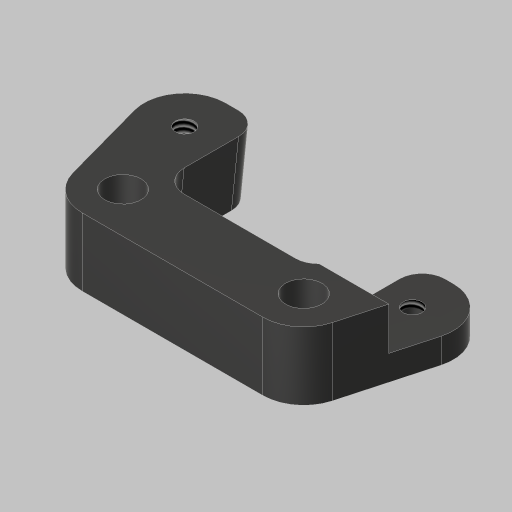
# Autodesk Inventor part: AR-020
Saved by Autodesk Inventor 2023.5 (Build 275446000, 446)
## iProperties
Created: 2025-02-28
Part Number: AR-020
Material: ABS Plastic
Document SubType Name: Modeling
Designer: brand
Density: 1.06 g/cm^3
Appearance: Smooth - Black
Author: brand
Autodesk Inventor part; units mm, degrees
ref_plane "YZ Plane" through (0, 0, 0) normal (1, 0, 0) x (0, 1, 0)
ref_plane "XZ Plane" through (0, 0, 0) normal (0, 1, 0) x (-1, 0, 0)
ref_plane "XY Plane" through (0, 0, 0) normal (0, 0, 1) x (1, 0, 0)
sketch "Sketch1" plane through (0, 0, 0) normal (0, 1, 0) x (-1, 0, 0)
  circle A0 centre (0, 0) radius 14.351 construction
  line L0 (-12.7, -34.925) -> (12.7, -34.925) construction
  circle A1 centre (0, 0) radius 22.225 construction
  circle A2 centre (0, 0) radius 31.75 construction
  circle A3 centre (-15.875, -27.4963) radius 4.7625 construction
  arc A4 (-20.4289, -28.8903) -> (-25.4478, -18.9862) centre (-51.4511, -38.3868) ccw construction
  arc A5 (-3.7186, -31.5315) -> (-14.8053, -32.1371) centre (-7.5184, -63.7513) ccw construction
  line L1 (0, 0) -> (0, -22.225) construction
  circle A6 centre (15.875, -27.4963) radius 4.7625 construction
  arc A7 (25.4478, -18.9862) -> (20.4289, -28.8903) centre (51.4511, -38.3868) ccw construction
  arc A8 (14.8053, -32.1371) -> (3.7186, -31.5315) centre (7.5184, -63.7513) ccw construction
  circle A9 centre (-12.7, -34.925) radius 2.5527 construction
  circle A10 centre (-12.7, -34.925) radius 3.1548 construction
  circle A11 centre (12.7, -34.925) radius 3.1548 construction
  line L2 (-16, -53.9) -> (16, -53.9) construction
  circle A12 centre (0, 0) radius 53.9 construction
  circle A13 centre (0, -40.64) radius 2.5527 construction
  circle A14 centre (12.7, -41.91) radius 2.5527 construction
  point P0 (0, -34.925)
  point P1 (31.75, 0)
  point P2 (15.875, 27.4963)
  point P3 (-15.875, 27.4963)
  point P4 (-31.75, 0)
  point P5 (15.875, -27.4963)
  point P6 (0, -53.9)
  point P7 (0, -53.9)
  point P8 (-12.7, -41.91)
  dimension "d3" = 44.45
  dimension "d16" = 107.8
  dimension "d0" = 28.702
  dimension "d1" = 25.4
  dimension "d2" = 34.925
  dimension "d4" = 63.5
  dimension "d7" = 360
  dimension "d9" = 9.525
  dimension "d10" = 32.4431
  dimension "d11" = 32.4431
  dimension "d12" = 5.1054
  dimension "d14" = 0.6021
  dimension "d15" = 32
  dimension "d18" = 40.64
  dimension "d19" = 5.1054
  dimension "d20" = 6.985
  dimension "d21" = 5.1054
  constraints: 15 point on circle, 13 centre point, 11 coincident, 7 symmetric about line, 7 vertical alignment, 6 end point, 6 tangent, 2 horizontal, 2 horizontal alignment, 2 midpoint, 1 vertical, 14 other
  measures "d0" diameter of A0
  measures "d1" distance of L0.start L0.end
  measures "d2" distance of point (0, 0) point (0, -34.925)
  measures "d4" diameter of A2
  measures "d9" diameter of A3
  measures "d10" radius of A4
  measures "d11" radius of A5
  measures "d12" diameter of A9
  measures "d14" radial gap between concentric circles of A10 A9
  measures "d15" distance of L2.start L2.end
  measures "d18" distance of point (0, 0) point (0, -40.64)
  measures "d19" diameter of A13
  measures "d20" distance from line of L0 point (-12.7, -41.91)
  measures "d21" diameter of A14
sketch "Sketch2" plane through (0, 0, 0) normal (0, 1, 0) x (-1, 0, 0)
  circle A0 centre (12.7, -41.91) radius 2.5527 construction
  circle A1 centre (12.7, -41.91) radius 5.7277 construction
  circle A2 centre (16, -53.9) radius 5.7277 construction
  line L0 (18.2224, -40.3901) -> (21.5224, -52.3801)
  circle A3 centre (-12.7, -41.91) radius 5.7277 construction
  circle A4 centre (-16, -53.9) radius 5.7277 construction
  line L1 (12.7, -36.1823) -> (-12.7, -36.1823)
  line L2 (-18.2224, -40.3901) -> (-21.5224, -52.3801)
  line L3 (-16, -59.6277) -> (16, -59.6277)
  arc A5 (18.2224, -40.3901) -> (12.7, -36.1823) centre (12.7, -41.91) ccw
  arc A6 (16, -59.6277) -> (21.5224, -52.3801) centre (16, -53.9) ccw
  arc A7 (-21.5224, -52.3801) -> (-16, -59.6277) centre (-16, -53.9) ccw
  arc A8 (-12.7, -36.1823) -> (-18.2224, -40.3901) centre (-12.7, -41.91) ccw
  line L4 (-12, -59.6277) -> (-12, -44.1197) construction
  line L5 (-12, -44.1197) -> (12, -44.1197) construction
  line L6 (12, -44.1197) -> (12, -59.6277) construction
  line L7 (12, -59.6277) -> (-12, -59.6277)
  line L8 (11, -44.1197) -> (-11, -44.1197)
  line L9 (-11, -44.1197) -> (-12, -59.6277)
  line L10 (11, -44.1197) -> (12, -59.6277)
  point P0 (0, 0)
  point P1 (0, -59.6277)
  point P2 (12, -59.6277)
  point P3 (0, -44.1197)
  point P4 (0, -44.1197)
  point P5 (12, -59.6277)
  dimension "d22" = 5.1054
  dimension "d23" = 3.175
  dimension "d40" = 24
  dimension "d41" = 15.508
  dimension "d45" = 22
  constraints: 22 end point, 16 point on circle, 9 centre point, 9 coincident, 7 tangent, 4 midpoint, 3 equal radius, 3 perpendicular, 2 point on line, 1 horizontal, 1 vertical
  measures "d22" diameter of A0
  measures "d23" radial gap between concentric circles of A0 A1
  measures "d40" distance of L4.end L5.end
  measures "d41" distance of L4.start L4.end
  measures "d45" distance of L8.end L8.start
extrude "Extrusion1" add sketch "Sketch2" against normal blind 9.525
hole "Hole1" at (-12.7, 0, -41.91) at (12.7, 0, -41.91) direction (0, -1, 0) diameter 5.1054 end through all clearance for "Flat Head Machine Screw (82)" size "#10" standard "Ansi Unified Screw Threads"
hole "Hole2" at (16, 0, -53.9) at (-16, 0, -53.9) direction (0, -1, 0) diameter 2.6416 end through all thread size "6-32 UNC" class "2B" standard "ANSI Unified Screw Threads"
sketch "Sketch3" plane through (0, -9.525, 0) normal (0, -1, 0) x (1, 0, 0)
  point P0 (0, 0)
sketch "Sketch4" plane through (16, 0, -59.6277) normal (0, 0, -1) x (-1, 0, 0)
  line L0 (28.7, 0) -> (3.3, 0) construction
  line L1 (5, 0) -> (27, 0)
  line L2 (27, 0) -> (28, -9.525)
  line L3 (28, -9.525) -> (4, -9.525)
  line L4 (3.3, -9.525) -> (28.7, -9.525) construction
  line L5 (4, -9.525) -> (5, 0)
  point P0 (16, 0)
  point P1 (16, 0)
  point P2 (16, -9.525)
  point P3 (16, -9.525)
  dimension "d46" = 22
  dimension "d47" = 24
  constraints: 8 end point, 4 midpoint, 4 point on line, 1 coincident
  measures "d46" distance of L1.end L1.start
  measures "d47" distance of L2.end L3.end
extrude "Extrusion3" cut sketch "Sketch4" against normal blind 14
fillet "Fillet2" radius 3.175 4 edges at (11.5, -4.7625, -45.6277) (-11.5, -4.7625, -45.6277) (-11.5, -4.7625, -59.6277) (11.5, -4.7625, -59.6277)
sketch "Sketch5" plane through (0, 0, 0) normal (1, 0, 0) x (0, 1, 0)
  line L0 (-9.525, -45.6277) -> (-9.525, -36.1823) construction
  line L1 (-9.525, -36.1823) -> (0, -36.1823) construction
  line L2 (0, -36.1823) -> (0, -45.6277) construction
  line L3 (0, -45.6277) -> (-9.525, -45.6277) construction
  line L4 (0, -59.6277) -> (-6, -59.6277)
  line L5 (-6, -59.6277) -> (-6, -46.6277)
  line L6 (-6, -46.6277) -> (0, -46.6277)
  line L7 (0, -46.6277) -> (0, -59.6277)
  line L8 (-9.525, -59.6277) -> (0, -59.6277) construction
  line L9 (-9.525, -56.4527) -> (-9.525, -48.8027) construction
  point P0 (0, 0)
  dimension "d55" = 6
  dimension "d56" = 13
  constraints: 8 end point, 2 parallel, 1 horizontal, 1 perpendicular
  measures "d55" distance from line of L5 L4.start
  measures "d56" distance of L4.end L5.end
extrude "Extrusion4" cut sketch "Sketch5" along normal blind 25.4
equation "\"d11\" = d10"
body "Solid1"
